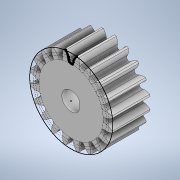
# Autodesk Inventor part: vertical_axis_small_gear
Saved by Autodesk Inventor 2021 (Build 250183000, 183)
## iProperties
Created: 2020-10-03
Part Number: vertical_axis_small_gear
Material: Generic
Document SubType Name: Modeling
Designer: bober
Density: 1 g/cm^3
Appearance: Default
Author: bober
Autodesk Inventor part; units mm, degrees
ref_plane "YZ Plane" through (0, 0, 0) normal (1, 0, 0) x (0, 1, 0)
ref_plane "XZ Plane" through (0, 0, 0) normal (0, 1, 0) x (-1, 0, 0)
ref_plane "XY Plane" through (0, 0, 0) normal (0, 0, 1) x (1, 0, 0)
sketch "Sketch1" plane through (0, 0, 0) normal (0, 0, 1) x (1, 0, 0)
  spline S0 degree 3 poles (-1.4753, 10.9006) (-1.4303, 10.8439) (-1.3402, 10.7303) (-1.214, 10.5533) (-1.0952, 10.3712) (-0.9853, 10.1836) (-0.8856, 9.9903) (-0.8127, 9.8244) (-0.7618, 9.6887) (-0.7284, 9.5853) (-0.6993, 9.4805) (-0.6881, 9.4089) (-0.6825, 9.3731) knots 0 0 0 0 0.125009 0.250018 0.375025 0.500029 0.62503 0.750024 0.812529 0.875031 0.93753 1 1 1 1
  spline S1 degree 3 poles (-0.6825, 9.3731) (-0.6788, 9.3211) (-0.6734, 9.243) (-0.6577, 9.1399) (-0.6419, 9.0633) (-0.6205, 8.9881) (-0.5955, 8.9139) (-0.5642, 8.8421) (-0.5257, 8.774) (-0.4815, 8.7093) (-0.4295, 8.6508) (-0.3703, 8.5994) (-0.304, 8.5574) (-0.2441, 8.5315) (-0.1945, 8.5152) (-0.156, 8.5084) (-0.1173, 8.502) (-0.0651, 8.501) (0, 8.5018) (0.0651, 8.501) (0.1173, 8.502) (0.156, 8.5084) (0.1945, 8.5152) (0.2441, 8.5315) (0.304, 8.5574) (0.3703, 8.5994) (0.4295, 8.6508) (0.4815, 8.7093) (0.5257, 8.774) (0.5642, 8.8421) (0.5955, 8.9139) (0.6205, 8.9881) (0.6419, 9.0633) (0.6577, 9.1399) (0.6734, 9.243) (0.6788, 9.3211) (0.6825, 9.3731) knots 0 0 0 0 0.062506 0.093766 0.125027 0.156286 0.187537 0.218798 0.250047 0.281288 0.312529 0.343769 0.374996 0.406221 0.421852 0.437476 0.453107 0.46874 0.5 0.53126 0.546893 0.562524 0.578148 0.593779 0.625004 0.656231 0.687471 0.718712 0.749953 0.781202 0.812463 0.843714 0.874973 0.906234 0.937494 1 1 1 1
  spline S2 degree 3 poles (0.6825, 9.3731) (0.6881, 9.4089) (0.6993, 9.4805) (0.7284, 9.5853) (0.7618, 9.6887) (0.8127, 9.8244) (0.8856, 9.9903) (0.9853, 10.1836) (1.0952, 10.3712) (1.214, 10.5533) (1.3402, 10.7303) (1.4303, 10.8439) (1.4753, 10.9006) knots 0 0 0 0 0.06247 0.124969 0.187471 0.249976 0.37497 0.499971 0.624975 0.749982 0.874991 1 1 1 1
  circle A0 centre (0, 0) radius 8.5015 construction
  circle A1 centre (0, 0) radius 9.3969 construction
  circle A2 centre (0, 0) radius 10 construction
  circle A3 centre (0, 0) radius 11
  point P0 (-1.3417, 10.7292)
  point P1 (-1.2152, 10.5524)
  point P2 (-1.0967, 10.3703)
  point P3 (-0.987, 10.1826)
  point P4 (-0.8877, 9.9894)
  point P5 (-0.8006, 9.7903)
  point P6 (-0.7626, 9.6885)
  point P7 (-0.7291, 9.5851)
  point P8 (-0.7013, 9.48)
  point P9 (-0.6688, 9.2173)
  point P10 (-0.6571, 9.14)
  point P11 (-0.641, 9.0635)
  point P12 (-0.6199, 8.9882)
  point P13 (-0.5945, 8.9143)
  point P14 (-0.563, 8.8427)
  point P15 (-0.5247, 8.7746)
  point P16 (-0.4802, 8.7103)
  point P17 (-0.4283, 8.652)
  point P18 (-0.3691, 8.6009)
  point P19 (-0.3031, 8.5592)
  point P20 (-0.2316, 8.5278)
  point P21 (-0.1943, 8.5161)
  point P22 (-0.156, 8.5085)
  point P23 (-0.1173, 8.5029)
  point P24 (-0.0782, 8.5014)
  point P25 (0, 8.5015)
  point P26 (0.0782, 8.5014)
  point P27 (0.1173, 8.5029)
  point P28 (0.156, 8.5085)
  point P29 (0.1943, 8.5161)
  point P30 (0.2316, 8.5278)
  point P31 (0.3031, 8.5592)
  point P32 (0.3691, 8.6009)
  point P33 (0.4283, 8.652)
  point P34 (0.4802, 8.7103)
  point P35 (0.5247, 8.7746)
  point P36 (0.563, 8.8427)
  point P37 (0.5945, 8.9143)
  point P38 (0.6199, 8.9882)
  point P39 (0.641, 9.0635)
  point P40 (0.6571, 9.14)
  point P41 (0.6688, 9.2173)
  point P42 (0.7013, 9.48)
  point P43 (0.7291, 9.5851)
  point P44 (0.7626, 9.6885)
  point P45 (0.8006, 9.7903)
  point P46 (0.8877, 9.9894)
  point P47 (0.987, 10.1826)
  point P48 (1.0967, 10.3703)
  point P49 (1.2152, 10.5524)
  point P50 (1.3417, 10.7292)
  constraints: 4 centre point, 2 point on circle, 117 other
extrude "Extrusion1" add sketch "Sketch1" against normal blind 10
extrude "Extrusion2" cut sketch "Sketch1" against normal blind 10 contours A3 S2 S1 S0 picked at (0.1626, 10.2155)
pattern_circular "Circular Pattern1" count 20 over 360 about axis through (0, 0, 0) along (0, 0, -1) of "Extrusion2"
hole "Hole1" at (0, 0, 0) direction (0, 0, -1) diameter 4.9 end through all
sketch "Sketch2" plane through (0, 0, 0) normal (0, 0, 1) x (1, 0, 0)
  point P0 (0, 0)
sketch "Sketch3" plane through (0, 0, 0) normal (0, 0, 1) x (1, 0, 0)
  point P0 (0, 0)
sketch "Sketch4" plane through (0, 0, 0) normal (0, 0, 1) x (1, 0, 0)
  circle A0 centre (0, 0) radius 2.45 projected
  line L0 (2.0954, 1.2696) -> (2.0954, -1.2696)
  line L1 (2.0954, 1.2696) -> (3.5793, 1.2696)
  line L2 (3.5793, 1.2696) -> (3.5793, -1.3346)
  line L3 (3.5793, -1.3346) -> (2.0954, -1.3346)
  line L4 (2.0954, -1.3346) -> (2.0954, 1.2696)
  point P0 (2.0546, -1.3346)
  point P1 (2.0954, -1.2696)
  constraints: 10 end point, 2 parallel, 2 point on circle, 1 horizontal, 1 perpendicular, 1 vertical
extrude "Extrusion3" add sketch "Sketch4" against normal blind 10 contours A0 L0 | A0 L1 L2 L3 L4 picked at (2.1603, -0.2901)
equation "\"d0\" = FaceWidth"
equation "\"Module\" = 1"
equation "\"PressureAngle\" = 20deg"
equation "\"UnitProfileClearance\" = 0.25"
equation "\"UnitRoundRadius\" = 0.35"
equation "\"HeadDiameter\" = 22"
equation "\"RootDiameter\" = 17.00295"
equation "\"BaseDiameter\" = 18.79385"
equation "\"FaceWidth\" = 10"
equation "\"HelixAngle\" = 0"
equation "\"UnitCorrection\" = 0"
equation "\"UnitAddendumModification\" = 0"
equation "\"CircularPitch\" = 3.141593"
equation "\"UnitBacklashShift\" = -0.248523"
equation "\"TotalToolShift\" = -0.24852"
equation "\"IsInternal\" = 0"
body "Solid1"
